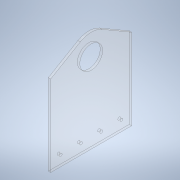
# Autodesk Inventor part: Jeep Plate 2.1
Saved by Autodesk Inventor 2020 (Build 240168000, 168)
## iProperties
Created: 2020-02-14
Part Number: Jeep Plate 2.1
Material: Polycarbonate, Clear
Document SubType Name: Modeling
Designer: aidan
Density: 1.2 g/cm^3
Appearance: Polycarbonate - Clear
Author: aidan
Autodesk Inventor part; units mm, degrees
ref_plane "YZ Plane" through (0, 0, 0) normal (1, 0, 0) x (0, 1, 0)
ref_plane "XZ Plane" through (0, 0, 0) normal (0, 1, 0) x (-1, 0, 0)
ref_plane "XY Plane" through (0, 0, 0) normal (0, 0, 1) x (1, 0, 0)
sketch "Sketch1" plane through (0, 0, 0) normal (1, 0, 0) x (0, 1, 0)
  line L0 (127, 101.6) -> (0, 101.6)
  line L1 (0, 101.6) -> (0, 0)
  line L2 (0, 0) -> (127, 0)
  line L3 (127, 0) -> (127, 101.6)
  circle A0 centre (100.0125, 50.8) radius 14.2875
  circle A1 centre (100.0125, 50.8) radius 26.9875
  line L4 (123.3175, 64.4088) -> (101.6, 101.6)
  line L5 (123.3175, 37.1912) -> (101.6, 0)
  dimension "d0" = 101.6
  dimension "d1" = 127
  dimension "d2" = 12.7
  dimension "d3" = 50.8
  dimension "d5" = 28.575
  dimension "d6" = 101.6
  dimension "d7" = 101.6
  constraints: 12 end point, 3 tangent, 2 centre point, 2 coincident, 2 parallel, 2 point on circle, 2 point on line, 1 horizontal, 1 perpendicular
  measures "d0" distance of L0.end L1.end
  measures "d1" distance of L1.end L2.end
  measures "d2" radial gap between concentric circles of A0 A1
  measures "d3" distance from line of L0 A0.centre
  measures "d5" diameter of A0
  measures "d6" distance from line of L1 L5.end
  measures "d7" distance from line of L1 L4.end
extrude "Extrusion1" add sketch "Sketch1" along normal blind 2.9972 contours L4 A1 L5 L2 L1 L0 | A1
sketch "Sketch2" plane through (2.9972, 0, 0) normal (1, 0, 0) x (0, 0, -1)
  circle A0 centre (-88.9, 12.7) radius 1.7272
  line L0 (-101.6, 101.6) -> (-101.6, 0) projected
  line L1 (-101.6, 0) -> (0, 0) projected
  dimension "d10" = 12.7
  dimension "d11" = 12.7
  dimension "d12" = 3.4544
  constraints: 1 centre point
  measures "d10" distance from line of L0 A0.centre
  measures "d11" distance from line of L1 A0.centre
  measures "d12" diameter of A0
extrude "Extrusion2" cut sketch "Sketch2" against normal blind 2.9972
pattern_linear "Rectangular Pattern1" count 4 spacing 25.4 along (0, 0, -1) of "Extrusion2"
body "Solid1"
